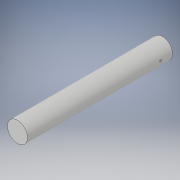
# Autodesk Inventor part: OuterRadiusPoleAJB
Saved by Autodesk Inventor 2018 (Build 220112000, 112)
## iProperties
Created: 2018-02-02
Part Number: OuterRadiusPoleAJB
Material: Generic
Document SubType Name: Modeling
Designer: Alec temporary
Density: 1 g/cm^3
Appearance: Default
Author: Alec temporary
Autodesk Inventor part; units mm, degrees
ref_plane "XZ Plane" through (0, 0, 0) normal (0, 1, 0) x (-1, 0, 0)
ref_plane "XY Plane" through (0, 0, 0) normal (0, 0, 1) x (1, 0, 0)
sketch "Sketch1" plane through (0, 0, 0) normal (0, 0, 1) x (1, 0, 0)
  circle A0 centre (0, 0) radius 127
  dimension "d0" = 254
  constraints: 1 centre point, 1 coincident
  measures "d0" diameter of A0
extrude "Extrusion1" add sketch "Sketch1" along normal blind 1828.8
ref_plane "Work Plane1" through (-127, 0, 0) normal (1, 0, 0) x (0, 1, 0)
sketch "Sketch2" plane through (0, 0, 0) normal (0, 0, -1) x (-1, 0, 0)
  circle A0 centre (0, 0) radius 101.6
  dimension "d3" = 203.2
  constraints: 1 centre point, 1 coincident
  measures "d3" diameter of A0
extrude "Extrusion2" cut sketch "Sketch2" against normal blind 304.8
sketch "Sketch3" plane through (-127, 0, 0) normal (1, 0, 0) x (0, 1, 0)
  circle A0 centre (0, 152.4) radius 12.7
  point P0 (0, 0)
  dimension "d6" = 25.4
  dimension "d7" = 152.4
  constraints: 1 centre point, 1 vertical alignment
  measures "d6" diameter of A0
  measures "d7" distance of point (0, 0) A0.centre
hole "Hole1" at (-127, 0, 152.4) direction (1, 0, 0) diameter 21.971 end through all thread size "1-8 UNC" class "2B" standard "ANSI Unified Screw Threads"
body "Solid1"
